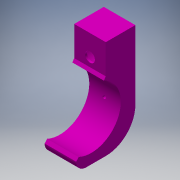
# Autodesk Inventor part: support-moteur
Saved by Autodesk Inventor 2017 (Build 210142000, 142)
## iProperties
Created: 2018-03-31
Part Number: support-moteur
Material: Generic
Document SubType Name: Modeling
Designer: franc
Density: 1 g/cm^3
Appearance: Default
Author: franc
Autodesk Inventor part; units mm, degrees
ref_plane "YZ Plane" through (0, 0, 0) normal (1, 0, 0) x (0, 1, 0)
ref_plane "XZ Plane" through (0, 0, 0) normal (0, 1, 0) x (-1, 0, 0)
ref_plane "XY Plane" through (0, 0, 0) normal (0, 0, 1) x (1, 0, 0)
sketch "Esquisse1" plane through (0, 0, 0) normal (0, 1, 0) x (-1, 0, 0)
  line L0 (14.0671, 6.9597) -> (-17.9329, 6.9597)
  line L1 (-17.9329, 6.9597) -> (-17.9329, -18.0403)
  line L2 (-17.9329, -18.0403) -> (14.0671, -18.0403)
  line L3 (14.0671, -18.0403) -> (14.0671, 6.9597)
  point P0 (0, 0)
  dimension "d0" = 25
  dimension "d1" = 32
  constraints: 8 end point, 2 parallel, 1 horizontal, 1 perpendicular
  measures "d0" distance of L2.end L0.start
  measures "d1" distance of L1.end L2.end
extrude "Extrusion1" add sketch "Esquisse1" along normal blind 30
sketch "Esquisse2" plane through (0, 30, 0) normal (0, 1, 0) x (1, 0, 0)
  circle A0 centre (1.9329, 9.0403) radius 15
  line L0 (-14.0671, 18.0403) -> (-14.0671, -6.9597) projected
  line L1 (-14.0671, -6.9597) -> (17.9329, -6.9597) projected
  point P0 (0, 0)
  dimension "d4" = 30
  dimension "d5" = 16
  dimension "d6" = 16
  constraints: 1 centre point
  measures "d4" diameter of A0
  measures "d5" distance from line of L0 A0.centre
  measures "d6" distance from line of L1 A0.centre
extrude "Extrusion2" cut sketch "Esquisse2" against normal blind 28
sketch "Esquisse3" plane through (1.9329, 2, -9.0403) normal (0, 1, 0) x (1, 0, 0)
  circle A0 centre (0, 0) radius 5
  line L0 (16, 9) -> (-16, 9) projected
  line L1 (-16, 9) -> (-16, -16) projected
  line L2 (-16, -16) -> (16, -16) projected
  point P0 (-1.9329, -9.0403)
  dimension "d9" = 10
  dimension "d11" = 16
  dimension "d14" = 16
  constraints: 1 centre point
  measures "d9" diameter of A0
  measures "d11" distance from line of L1 A0.centre
  measures "d14" distance from line of L2 A0.centre
extrude "Extrusion3" cut sketch "Esquisse3" against normal through all
sketch "Esquisse5" plane through (17.9329, 0, -18.0403) normal (0, 0, -1) x (-1, 0, 0)
  line L0 (28, 30) -> (28, 2) projected
  line L1 (32, 30) -> (28, 30)
  line L2 (28, 30) -> (28, 16)
  line L3 (28, 16) -> (32, 16)
  line L4 (32, 16) -> (32, 30)
  line L5 (28, 30) -> (32, 30) projected
  line L6 (32, 0) -> (32, 30) projected
  line L7 (4, 2) -> (4, 30) projected
  line L8 (0, 30) -> (4, 30) projected
  line L9 (4, 16) -> (0, 16)
  line L10 (0, 16) -> (0, 30)
  line L11 (0, 30) -> (4, 30)
  line L12 (4, 30) -> (4, 16)
  point P0 (17.9329, 0)
  dimension "d15" = 14
  dimension "d16" = 0
  dimension "d17" = 0
  dimension "d18" = 14
  constraints: 16 end point, 4 parallel, 2 horizontal, 2 midpoint, 2 perpendicular
  measures "d15" distance of L3.end L1.start
  measures "d16" distance between parallel lines of L5 L1
  measures "d17" distance between parallel lines of L6 L4
  measures "d18" distance of L9.end L8.start
extrude "Extrusion4" add sketch "Esquisse5" along normal blind 10
sketch "Esquisse6" plane through (17.9329, 0, -28.0403) normal (0, 0, -1) x (-1, 0, 0)
  line L0 (32, 16) -> (28, 16) projected
  line L1 (32, 30) -> (0, 30) projected
  line L2 (32, 16) -> (0, 16)
  line L3 (0, 16) -> (0, 30)
  line L4 (0, 30) -> (32, 30)
  line L5 (32, 30) -> (32, 16)
  point P0 (17.9329, 0)
  constraints: 8 end point, 2 parallel, 1 horizontal, 1 perpendicular
extrude "Extrusion5" add sketch "Esquisse6" along normal blind 50
sketch "Esquisse7" plane through (17.9329, 0, -78.0403) normal (0, 0, -1) x (-1, 0, 0)
  line L0 (32, 30) -> (0, 30) projected
  line L1 (32, 30) -> (0, 30)
  line L2 (0, 30) -> (0, -30)
  line L3 (0, -30) -> (32, -30)
  line L4 (32, -30) -> (32, 30)
  point P0 (17.9329, 0)
  dimension "d23" = 60
  constraints: 8 end point, 2 parallel, 1 horizontal, 1 perpendicular
  measures "d23" distance of L1.end L2.end
extrude "Extrusion6" add sketch "Esquisse7" along normal blind 10
sketch "Esquisse8" plane through (17.9329, 0, 6.9597) normal (1, 0, 0) x (0, 0, -1)
  ellipse E0 centre (54.9571, -14.73) end of major axis (54.9571, -44.73) minor radius 29.9996 projected
  ellipse E1 centre (54.9571, -14.73) end of major axis (54.9571, 12.27) minor radius 26.9996 projected
  ellipse E2 centre (54.9571, -14.73) end of major axis (54.9571, -44.73) minor radius 29.9996 projected
  arc A0 (82.092, -27.5236) -> (27.8222, -1.9363) centre (54.9571, -14.73) ccw
  line L0 (85, 16) -> (85, -30) projected
  line L1 (82.092, -27.5236) -> (85, -30)
  line L2 (25, 16) -> (85, 16) projected
  line L3 (85, -30) -> (85, 16)
  line L4 (85, 16) -> (25, 16)
  line L5 (25, 0) -> (25, 16) projected
  line L6 (25, 16) -> (25, 0)
  line L7 (25, 0) -> (27.8222, -1.9363)
  point P0 (6.9597, 0)
  constraints: 11 end point, 2 perpendicular, 2 point on circle, 1 centre point, 1 coincident, 1 collinear, 5 other
extrude "Extrusion7" add sketch "Esquisse8" against normal blind 32 contours E0 L7 L5 L2 L0 L1
fillet "Congé1" radius 30 1 edges at (1.9329, 30, -88.0403)
fillet "Congé2" radius 10 1 edges at (1.9329, -30, -88.0403)
sketch "Esquisse9" plane through (-10.0671, 16, -28.0403) normal (0, 1, 0) x (1, 0, 0)
  circle A0 centre (12, -19) radius 5 projected
  line L0 (0, -10) -> (24, -10) projected
  arc A1 (0, -10) -> (24, -10) centre (12, -19) ccw projected
  circle A2 centre (12, -19) radius 15
  point P0 (10.0671, -28.0403)
  dimension "d30" = 30
  constraints: 1 centre point, 1 coincident
  measures "d30" diameter of A2
extrude "Extrusion8" cut sketch "Esquisse9" against normal up to surface (14 mm away) contours A2 L0
sketch "Esquisse10" plane through (-14.0671, 0, 6.9597) normal (0, 0, 1) x (1, 0, 0)
  line L0 (32, 15.27) -> (32, -27.5236) projected
  line L1 (0, 30) -> (32, 30)
  line L2 (32, 30) -> (32, 0)
  line L3 (32, 0) -> (0, 0)
  line L4 (0, 0) -> (0, 30)
  point P0 (14.0671, 0)
  point P1 (32, -1.9363)
  constraints: 8 end point, 2 parallel, 1 horizontal, 1 perpendicular, 1 point on line
extrude "Extrusion9" add sketch "Esquisse10" along normal blind 5
sketch "Esquisse11" plane through (0, 30, 0) normal (0, 1, 0) x (1, 0, 0)
  circle A0 centre (1.3437, 52.0208) radius 1.5 projected
  point P0 (0, 0)
extrude "Extrusion10" cut sketch "Esquisse11" against normal through all
